Autodesk Fusion 360 part; units mm, degrees
(part 3 of 6)
sketch "Servo Holder" plane through (0, 0, 0) normal (0, 0, -1) x (1, 0, 0)
  line L0 (113.5, 9) -> (83.5, 9)
  line L1 (83.5, 9) -> (83.5, 39)
  line L2 (83.5, 39) -> (33.5, 39)
  arc A0 (33.5, 39) -> (18.5, 24) centre (33.5, 24) ccw
  arc A1 (18.5, 24) -> (22.1849, 0) centre (98.5, 24) ccw
  line L3 (22.1849, 0) -> (0, 0)
  line L4 (0, 0) -> (0, -76)
  line L5 (0, -76) -> (120, -76)
  line L6 (120, -76) -> (120, 0)
  line L7 (120, 0) -> (113.5, 0)
  line L8 (113.5, 0) -> (113.5, 9)
  circle A2 centre (32.5, 24) radius 9
  line L9 (120, 0) -> (79.5, 0)
  line L10 (79.5, 0) -> (79.5, 39)
  line L11 (79.5, 39) -> (120, 39)
  line L12 (120, 39) -> (120, 0)
  dimension "d192" = 40.5
  constraint horizontal L9
  constraint vertical L10
  constraint horizontal L11
  constraint vertical L12
  constraint coincident L6.end L7.start
  constraint collinear L2 L11
  measures "d192" distance of L10.end L11.end
extrude "Extrude46" add sketch "Servo Holder" along normal blind 29 contours L0 L1 L2 L8 L9 L10 L11 | L0 L1 L7 L8 L9 L11 L12
extrude "Extrude50" add 1 faces at (105.6667, -29, 0) along direction (0, 0, 1) blind 4
sketch "Servo Seat" plane through (0, 0, 4) normal (0, 0, 1) x (-1, 0, 0)
  line L0 (-113.5, -41) -> (-113.5, 9)
  line L1 (-113.5, 9) -> (-83.5, 9)
  line L2 (-83.5, 9) -> (-83.5, 39)
  line L3 (-83.5, 39) -> (-120, 39)
  line L4 (-120, 39) -> (-120, -76)
  line L5 (-120, -76) -> (0, -76)
  line L6 (0, -76) -> (0, 0)
  line L7 (0, 0) -> (-22.1849, 0)
  arc A0 (-98.5, -56) -> (-22.1849, 0) centre (-98.5, 24) ccw
  arc A1 (-113.5, -41) -> (-98.5, -56) centre (-98.5, -41) ccw
  line L8 (-83.5, 9) -> (-120, 9)
  line L9 (-120, 9) -> (-120, 18.5)
  line L10 (-120, 18.5) -> (-83.5, 18.5)
  line L11 (-83.5, 18.5) -> (-83.5, 9)
  line L12 (-83.5, 39) -> (-120, 39)
  line L13 (-120, 39) -> (-120, 30.5)
  line L14 (-120, 30.5) -> (-83.5, 30.5)
  line L15 (-83.5, 30.5) -> (-83.5, 39)
  line L16 (-120, 18.5) -> (-115, 18.5)
  line L17 (-115, 18.5) -> (-115, 30.5)
  line L18 (-115, 30.5) -> (-120, 30.5)
  line L19 (-120, 30.5) -> (-120, 18.5)
  line L20 (-113.5, 9) -> (-113.5, 18.5)
  line L21 (-113.5, 30.5) -> (-113.5, 39)
  dimension "d208" = 9.5
  dimension "d211" = 5
  dimension "d225" = 12
  dimension "d226" = 8.5
  dimension "d227" = 6.5
  constraint horizontal L8
  constraint vertical L9
  constraint horizontal L10
  constraint vertical L11
  constraint coincident L1.end L2.start
  constraint horizontal L12
  constraint vertical L13
  constraint horizontal L14
  constraint vertical L15
  constraint coincident L2.end L3.start
  constraint coincident L4 L9.end
  constraint horizontal L16
  constraint vertical L17
  constraint horizontal L18
  constraint vertical L19
  constraint coincident L14 L17.end
  constraint coincident L0.end L1.start
  constraint coincident L10 L20.end
  constraint perpendicular L10 L20
  constraint coincident L14 L21.start
  constraint coincident L3 L21.end
  constraint perpendicular L3 L21
  constraint collinear L20 L21
  constraint collinear L9 L13
  measures "d208" distance of L8.end L9.end
  measures "d211" distance of L17 L19
  measures "d225" distance of L9.end L13.end
  measures "d226" distance of L3.end L13.end
  measures "d227" distance of L13 L21
extrude "Extrude51" cut sketch "Servo Seat" against normal blind 13 contours L4 L10 L14 L16 L17 L18 L19
extrude "Extrude52" cut sketch "Servo Seat" against normal blind 4 contours L1 L2 L8 L10 L11 L20 | L2 L3 L12 L14 L15 L21
extrude "Extrude53" cut sketch "Servo Seat" against normal blind 29 contours L2 L10 L14 L17
sketch "Servo Wires Hole" plane through (79.5, 0, 0) normal (-1, 0, 0) x (0, -1, 0)
  line L0 (39, 0) -> (0, 0)
  line L1 (0, 0) -> (0, -29)
  line L2 (0, -29) -> (39, -29)
  line L3 (39, -29) -> (39, 0)
  line L4 (18.5, -15) -> (30.5, -15)
  line L5 (30.5, -15) -> (30.5, -25)
  line L6 (30.5, -25) -> (18.5, -25)
  line L7 (18.5, -25) -> (18.5, -15)
  dimension "d219" = 8.5
  dimension "d220" = 4
  dimension "d221" = 10
  dimension "d228" = 12
  constraint horizontal L4
  constraint vertical L5
  constraint horizontal L6
  constraint vertical L7
  measures "d219" distance of L3 L5
  measures "d220" distance of L2 L6
  measures "d221" distance of L4.end L5.end
  measures "d228" distance of L5.end L6.end
extrude "Extrude54" cut sketch "Servo Wires Hole" against normal blind 4 contours L4 L5 L6 L7
named bodies: "Colour Detection Mechanism Platform"

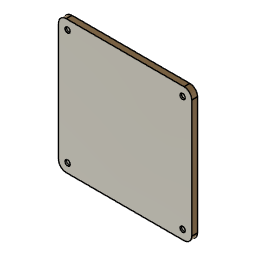
design "Bottom Access Panel"
Autodesk Fusion 360 part; units mm, degrees
sketch "Bottom Access Panel" plane through (0, 0, 0) normal (0, 1, 0) x (1, 0, 0)
  line L0 (0, 0) -> (139, 0)
  line L1 (139, 0) -> (139, -139)
  line L2 (139, -139) -> (0, -139)
  line L3 (0, -139) -> (0, 0)
  dimension "d1" = 139
  dimension "d2" = 139
  constraint horizontal L0
  constraint vertical L1
  constraint horizontal L2
  constraint vertical L3
  constraint coincident L0.start L3.end
  measures "d1" distance of L0.start L0.end
  measures "d2" distance of L0.end L1.end
extrude "Extrude1" add sketch "Bottom Access Panel" along normal blind 6
fillet "Fillet1" radius 8 4 edges at (0, 3, 139) (139, 3, 139) (139, 3, 0) (0, 3, 0)
sketch "Magnet Holes" plane through (0, 0, 0) normal (0, 1, 0) x (1, 0, 0)
  arc A0 (8, 0) -> (0, -8) centre (8, -8) ccw
  line L0 (8, 0) -> (131, 0)
  arc A1 (139, -8) -> (131, 0) centre (131, -8) ccw
  line L1 (139, -8) -> (139, -131)
  arc A2 (131, -139) -> (139, -131) centre (131, -131) ccw
  line L2 (131, -139) -> (8, -139)
  arc A3 (0, -131) -> (8, -139) centre (8, -131) ccw
  line L3 (0, -131) -> (0, -8)
  circle A4 centre (9.5, -129.5) radius 2.75
  circle A5 centre (129.5, -129.5) radius 2.75
  circle A6 centre (9.5, -9.5) radius 2.75
  circle A7 centre (129.5, -9.5) radius 2.75
  dimension "d20" = 5.5
  dimension "d21" = 5.5
  dimension "d22" = 5.5
  dimension "d23" = 5.5
  dimension "d24" = 9.5
  dimension "d25" = 9.5
  dimension "d26" = 9.5
  dimension "d27" = 9.5
  dimension "d28" = 9.5
  dimension "d29" = 9.5
  dimension "d30" = 9.5
  dimension "d31" = 9.5
  measures "d20" diameter of A4
  measures "d21" diameter of A5
  measures "d22" diameter of A6
  measures "d23" diameter of A7
  measures "d24" distance of L1 A5.centre
  measures "d25" distance of L2 A5.centre
  measures "d26" distance of L3 A4.centre
  measures "d27" distance of L2 A4.centre
  measures "d28" distance of L0 A6.centre
  measures "d29" distance of L3 A6.centre
  measures "d30" distance of L1 A7.centre
  measures "d31" distance of L0 A7.centre
extrude "Extrude3" cut sketch "Magnet Holes" along normal blind 1.5 contours A4 | A5 | A6 | A7
equation "mdfThickness = 6 mm"
equation "d4 = mdfThickness"
equation "filletRadius = 8 mm"
equation "d15 = filletRadius"
named bodies: "Bottom Access Panel"

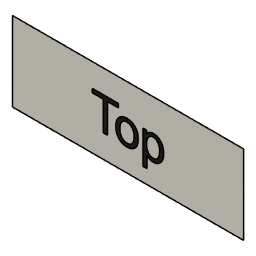
design "Top Label"
part number: 2025-04-13-09-56-45-957
Autodesk Fusion 360 part; units mm, degrees
sketch "Sticker" plane through (0, 0, 0) normal (0, 1, 0) x (1, 0, 0)
  line L0 (0, 0) -> (35, 0)
  line L1 (35, 0) -> (35, -12)
  line L2 (35, -12) -> (0, -12)
  line L3 (0, -12) -> (0, 0)
  dimension "d1" = 35
  dimension "d2" = 12
  constraint horizontal L0
  constraint vertical L1
  constraint horizontal L2
  constraint vertical L3
  constraint coincident L0.start L3.end
  measures "d1" distance of L0.start L0.end
  measures "d2" distance of L0.end L1.end
extrude "Extrude1" add sketch "Sticker" along normal blind 0.01 makes body 1
sketch "Text" plane through (0, 0, 0) normal (0, -1, 0) x (1, 0, 0)
  line L0 (35, 12) -> (0, 12)
  line L1 (0, 12) -> (0, 0)
  line L2 (0, 0) -> (35, 0)
  line L3 (35, 0) -> (35, 12)
  line L4 (0, 0) -> (35, 0) construction
  line L5 (35, 0) -> (35, 12) construction
  line L6 (35, 12) -> (0, 12) construction
  line L7 (0, 12) -> (0, 0) construction
  dimension "d5" = 5
  text T0 "Top" font "Arial" height 5 align centre middle in box 35 x 12 at (0, 0) x (1, 0) y (0, 1) spacing 1 kerned
  constraint coincident L2.end
  constraint coincident L0.end
extrude "Extrude2" add sketch "Text" along normal blind 0.01 separate body text T0 makes body 2 at (19.9566, 0, 4.7193) makes body 3 at (15.8803, 0, 5.5613) makes body 4 at (14.1792, 0, 4.97)
named bodies: "Sticker", "Text 3", "Text 2", "Text 1"

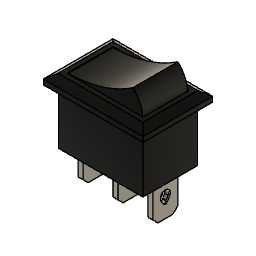
design "Power Switch"
Autodesk Fusion 360 part; units mm, degrees
sketch "Main body" plane through (0, 0, 0) normal (0, 0, 1) x (1, 0, 0)
  line L0 (0, 0) -> (17, 0)
  line L1 (17, 0) -> (17, 11)
  line L2 (17, 11) -> (0, 11)
  line L3 (0, 11) -> (0, 0)
  dimension "d1" = 17
  dimension "d2" = 11
  constraint horizontal L0
  constraint vertical L1
  constraint horizontal L2
  constraint vertical L3
  constraint coincident L0.start L3.end
  measures "d1" distance of L0.start L0.end
  measures "d2" distance of L0.end L1.end
extrude "Extrude1" add sketch "Main body" along normal blind 11 makes body 1
sketch "Top Plate" plane through (0, 0, 11) normal (0, 0, 1) x (-1, 0, 0)
  line L0 (0, -11) -> (0, 0)
  line L1 (0, 0) -> (-17, 0)
  line L2 (-17, 0) -> (-17, -11)
  line L3 (-17, -11) -> (0, -11)
  line L4 (1.5, -12.5) -> (-18.5, -12.5)
  line L5 (-18.5, -12.5) -> (-18.5, 1.5)
  line L6 (-18.5, 1.5) -> (1.5, 1.5)
  line L7 (1.5, 1.5) -> (1.5, -12.5)
  dimension "d5" = 20
  dimension "d6" = 1.5
  dimension "d7" = 1.5
  dimension "d8" = 14
  dimension "d9" = 1.5
  dimension "d10" = 1.5
  constraint horizontal L4
  constraint vertical L5
  constraint horizontal L6
  constraint vertical L7
  measures "d5" distance of L5.end L6.end
  measures "d6" distance of L0 L7
  measures "d7" distance of L2 L5
  measures "d8" distance of L4.end L5.end
  measures "d9" distance of L3 L4
  measures "d10" distance of L1 L6
extrude "Extrude2" add sketch "Top Plate" along normal blind 2 contours L0 L1 L2 L3 | L4 L5 L6 L7 bodies 1
chamfer "Chamfer1" distance 1.5 distance2 1 1 edges at (8.5, -1.5, 13) measured on face at (11.8333, 7.8333, 13) on bodies 1
chamfer "Chamfer1" distance 1.5 distance2 1 3 edges at (18.5, 5.5, 13) (8.5, 12.5, 13) (-1.5, 5.5, 13) measured on face at (11.8333, 7.8333, 13) measured on face at (11.8333, 7.8333, 13) measured on face at (11.8333, 7.8333, 13) on bodies 1
sketch "Switch" plane through (0, 0, 13) normal (0, 0, 1) x (-1, 0, 0)
  line L0 (-17, -11) -> (0, -11)
  line L1 (0, -11) -> (0, 0)
  line L2 (0, 0) -> (-17, 0)
  line L3 (-17, 0) -> (-17, -11)
  line L4 (-1, -10) -> (-16, -10)
  line L5 (-16, -10) -> (-16, -1)
  line L6 (-16, -1) -> (-1, -1)
  line L7 (-1, -1) -> (-1, -10)
  line L8 (-0.9, -10.1) -> (-16.1, -10.1)
  line L9 (-16.1, -10.1) -> (-16.1, -0.9)
  line L10 (-16.1, -0.9) -> (-0.9, -0.9)
  line L11 (-0.9, -0.9) -> (-0.9, -10.1)
  line L12 (-16, -10) -> (-14, -10)
  line L13 (-14, -10) -> (-14, -1)
  line L14 (-14, -1) -> (-16, -1)
  line L15 (-16, -1) -> (-16, -10)
  dimension "d17" = 1
  dimension "d18" = 1
  dimension "d19" = 1
  dimension "d20" = 1
  dimension "d21" = 0.1
  dimension "d22" = 0.1
  dimension "d23" = 0.1
  dimension "d24" = 0.1
  dimension "d29" = 2
  constraint horizontal L4
  constraint vertical L5
  constraint horizontal L6
  constraint vertical L7
  constraint horizontal L8
  constraint vertical L9
  constraint horizontal L10
  constraint vertical L11
  constraint horizontal L12
  constraint vertical L13
  constraint horizontal L14
  constraint vertical L15
  constraint coincident L6 L13.end
  measures "d17" distance of L0 L4
  measures "d18" distance of L2 L6
  measures "d19" distance of L1 L7
  measures "d20" distance of L3 L5
  measures "d21" distance of L4 L8
  measures "d22" distance of L6 L10
  measures "d23" distance of L7 L11
  measures "d24" distance of L5 L9
  measures "d29" distance of L5 L13
extrude "Extrude3" cut sketch "Switch" against normal blind 1 contours L8 L9 L10 L11 bodies 1
extrude "Extrude4" add sketch "Switch" along normal blind 4 contours L4 L5 L6 L12 L13 L14 L15 bodies 1
fillet "Fillet1" radius 6.25 1 edges at (16, 5.5, 17) on bodies 1
fillet "Fillet2" radius 23.5 1 edges at (14, 5.5, 13) on bodies 1
sketch "Pins" plane through (0, 0, 0) normal (0, 0, -1) x (1, 0, 0)
  line L0 (0, 0) -> (0, -11)
  line L1 (0, -11) -> (17, -11)
  line L2 (17, -11) -> (17, 0)
  line L3 (17, 0) -> (0, 0)
  line L4 (1, -8) -> (2, -8)
  line L5 (2, -8) -> (2, -3)
  line L6 (2, -3) -> (1, -3)
  line L7 (1, -3) -> (1, -8)
  line L8 (8, -8) -> (9, -8)
  line L9 (9, -8) -> (9, -3)
  line L10 (9, -3) -> (8, -3)
  line L11 (8, -3) -> (8, -8)
  line L12 (15, -8) -> (16, -8)
  line L13 (16, -8) -> (16, -3)
  line L14 (16, -3) -> (15, -3)
  line L15 (15, -3) -> (15, -8)
  dimension "d34" = 5
  dimension "d37" = 1
  dimension "d38" = 1
  dimension "d39" = 1
  dimension "d40" = 1
  dimension "d41" = 1
  dimension "d42" = 6
  dimension "d43" = 6
  dimension "d44" = 3
  dimension "d45" = 3
  constraint horizontal L4
  constraint vertical L5
  constraint horizontal L6
  constraint vertical L7
  constraint horizontal L8
  constraint vertical L9
  constraint horizontal L10
  constraint vertical L11
  constraint horizontal L12
  constraint vertical L13
  constraint horizontal L14
  constraint vertical L15
  constraint collinear L6 L10
  constraint collinear L10 L14
  constraint collinear L4 L8
  constraint collinear L8 L12
  measures "d34" distance of L4.start L6.end
  measures "d37" distance of L8.start L8.end
  measures "d38" distance of L4.start L4.end
  measures "d39" distance of L12.start L12.end
  measures "d40" distance of L2 L13
  measures "d41" distance of L0 L7
  measures "d42" distance of L5 L11
  measures "d43" distance of L9 L15
  measures "d44" distance of L3 L6
  measures "d45" distance of L1 L4
extrude "Extrude5" add sketch "Pins" along normal blind 7 separate body contours L4 L5 L6 L7 | L8 L9 L10 L11 | L12 L13 L14 L15 makes body 2 at (1, 4.6667, -2.3333) makes body 3 at (8, 4.6667, -2.3333) makes body 4 at (15, 4.6667, -2.3333)
chamfer "Chamfer2" distance 1 angle 45 6 edges at (1.5, 3, -7) (1.5, 8, -7) (15.5, 3, -7) (15.5, 8, -7) (8.5, 3, -7) (8.5, 8, -7) on bodies 2 3 4
sketch "Right Pin Hole" plane through (16, 0, 0) normal (1, 0, 0) x (0, 1, 0)
  line L0 (7, -7) -> (8, -6)
  line L1 (8, -6) -> (8, 0)
  line L2 (8, 0) -> (3, 0)
  line L3 (3, 0) -> (3, -6)
  line L4 (3, -6) -> (4, -7)
  line L5 (4, -7) -> (7, -7)
  circle A0 through (6.4999, -3, -0.005) (5.0001, -2.134, 0.0218) (5, -3.866, 0.0089)
  circle A1 through (6.0012, -4, -0.0057) (5.2512, -3.567, 0.0077) (5.2512, -4.433, 0.0013)
  line L6 (5.9345, -4.2494, -0.0066) -> (6.3666, -3.4989, -0.0069)
  line L7 (5.0685, -4.2505, 0.0052) -> (4.6347, -3.5011, 0.0166)
  dimension "d49" = 2
  dimension "d50" = 4
  dimension "d51" = 2.5
  dimension "d52" = 1
sketch "Middle Pine Hole" plane through (9, 0, 0) normal (1, 0, 0) x (0, 1, 0)
  line L0 (7, -7) -> (8, -6)
  line L1 (8, -6) -> (8, 0)
  line L2 (8, 0) -> (3, 0)
  line L3 (3, 0) -> (3, -6)
  line L4 (3, -6) -> (4, -7)
  line L5 (4, -7) -> (7, -7)
  ellipse E0 centre (5.5, -3) end of major axis (5.9789, -2.1221) minor radius 0.9999
  ellipse E1 centre (5.5012, -4) end of major axis (5.7406, -3.561) minor radius 0.4999
  line L6 (5.9345, -4.2494) -> (6.3666, -3.4989)
  line L7 (5.0685, -4.2505) -> (4.6347, -3.5011)
sketch "Left Pin Hole" plane through (2, 0, 0) normal (1, 0, 0) x (0, 1, 0)
  line L0 (7, -7) -> (8, -6)
  line L1 (8, -6) -> (8, 0)
  line L2 (8, 0) -> (3, 0)
  line L3 (3, 0) -> (3, -6)
  line L4 (3, -6) -> (4, -7)
  line L5 (4, -7) -> (7, -7)
  ellipse E0 centre (5.5, -3) end of major axis (5.9789, -2.1221) minor radius 0.9999
  line L6 (5.0685, -4.2505) -> (4.6347, -3.5011)
  ellipse E1 centre (5.5012, -4) end of major axis (5.7406, -3.561) minor radius 0.4999
  line L7 (5.9345, -4.2494) -> (6.3666, -3.4989)
extrude "Extrude6" cut sketch "Left Pin Hole" against normal blind 1 contours E0 E1 | E0 L6 E1 | E0 E1 L7 | E0 E1 | E0 E1 bodies 2
extrude "Extrude7" cut sketch "Middle Pine Hole" against normal blind 1 contours E0 E1 | E0 E1 L7 | E0 E1 L6 | E0 E1 | E0 E1 bodies 3
extrude "Extrude8" cut sketch "Right Pin Hole" against normal blind 1 contours A0 A1 | A0 A1 L7 | A0 A1 L6 | A0 A1 | A0 A1 in plane through (16.1055, 0.0014, -0.0008) normal (0.99988, 0.01358, -0.007407) bodies 4
equation "d6 = ( ( 20 - 17 ) / 2 ) * 1 mm"
equation "d9 = ( ( 14 - 11 ) / 2 ) * 1 mm"
equation "d44 = ( ( 11 - 5 ) / 2 ) * 1 mm"
named bodies: "Main Body", "Left Pin", "Middle Pin", "Right Pin"

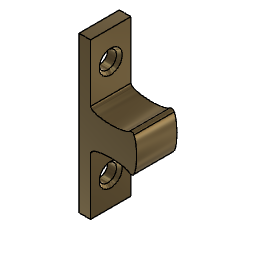
design "Clip Connector Clip"
Autodesk Fusion 360 part; units mm, degrees
sketch "Sketch1" plane through (0, 0, 0) normal (1, 0, 0) x (0, 1, 0)
  line L0 (0, 0) -> (7, 0)
  line L1 (7, 0) -> (7, 27)
  line L2 (7, 27) -> (0, 27)
  line L3 (0, 27) -> (0, 0)
  dimension "d1" = 7
  dimension "d2" = 27
  constraint horizontal L0
  constraint vertical L1
  constraint horizontal L2
  constraint vertical L3
  constraint coincident L0.start L3.end
  measures "d1" distance of L1.end L2.end
  measures "d2" distance of L0.end L1.end
extrude "Extrude1" add sketch "Sketch1" along normal blind 2
sketch "Sketch2" plane through (2, 0, 0) normal (1, 0, 0) x (0, 1, 0)
  line L0 (0, 27) -> (0, 0)
  line L1 (0, 0) -> (7, 0)
  line L2 (7, 0) -> (7, 27)
  line L3 (7, 27) -> (0, 27)
  line L4 (0, 17) -> (7, 17)
  line L5 (7, 17) -> (7, 10)
  line L6 (7, 10) -> (0, 10)
  line L7 (0, 10) -> (0, 17)
  circle A0 centre (3.5, 22) radius 1.5
  circle A1 centre (3.5, 5) radius 1.5
  dimension "d5" = 3.5
  dimension "d6" = 3.5
  dimension "d7" = 3
  dimension "d8" = 3
  dimension "d9" = 7
  dimension "d10" = 10
  dimension "d11" = 10
  dimension "d12" = 5
  dimension "d13" = 5
  dimension "d33" = 5
  dimension "d34" = 5
  constraint horizontal L4
  constraint vertical L5
  constraint horizontal L6
  constraint vertical L7
  constraint coincident L2 L5.end
  constraint coincident L0 L4.start
  measures "d5" distance of L0 A0.centre
  measures "d6" distance of L0 A1.centre
  measures "d7" diameter of A0
  measures "d8" diameter of A1
  measures "d9" distance of L4 L6
  measures "d10" distance of L3 L4
  measures "d11" distance of L1 L6
  measures "d12" distance of L3 A0.centre
  measures "d13" distance of L1 A1.centre
  measures "d33" distance of L4 A0.centre
  measures "d34" distance of L6 A1.centre
extrude "Extrude2" cut sketch "Sketch2" against normal blind 2 contours A0 | A1
chamfer "Chamfer1" distance 0.5 angle 45 2 edges at (2, 2.1015, 22.5424) (2, 2.1015, 5.5424)
extrude "Extrude3" add sketch "Sketch2" along normal blind 7 contours L0 L2 L4 L5 L6 L7
sketch "Sketch4" plane through (0, 0, 0) normal (0, -1, 0) x (1, 0, 0)
  line L0 (0, 27) -> (0, 0)
  line L1 (0, 0) -> (2, 0)
  line L2 (2, 0) -> (2, 10)
  line L3 (2, 10) -> (9, 10)
  line L4 (9, 10) -> (9, 17)
  line L5 (9, 17) -> (2, 17)
  line L6 (2, 17) -> (2, 27)
  line L7 (2, 27) -> (0, 27)
  ellipse E0 centre (9, 13.5) end of major axis (9, 17) minor radius 1
  line L8 (9, 10) -> (9, 17)
  line L9 (10, 13.5) -> (8, 13.5)
  dimension "d35" = 2
  constraint coincident L3.end E0
  constraint coincident L4.end E0
  constraint coincident E0 L9.start
  constraint coincident E0 L9.end
extrude "Extrude5" add sketch "Sketch4" against normal blind 7 contours L4 E0 L8 L9 | L4 E0 L8 L9 picked at (9.6303, 14.0297) picked at (9.2475, 11.5518)
sketch "Sketch5" plane through (0, 0, 0) normal (0, -1, 0) x (1, 0, 0)
  line L0 (0, 27) -> (0, 0)
  line L1 (0, 0) -> (2, 0)
  line L2 (2, 0) -> (2, 10)
  line L3 (2, 10) -> (9, 10)
  line L4 (9, 17) -> (2, 17)
  line L5 (2, 17) -> (2, 27)
  line L6 (2, 27) -> (0, 27)
  ellipse E0 centre (9, 13.5) end of major axis (9, 17) minor radius 1 (9, 10) -> (9, 17) ccw
  ellipse E1 centre (5.5, 17) end of major axis (9, 17) minor radius 1
  line L7 (2, 17) -> (9, 17)
  line L8 (5.5, 16) -> (5.5, 18)
  ellipse E2 centre (5.5, 10) end of major axis (9, 10) minor radius 1
  line L9 (2, 10) -> (9, 10)
  line L10 (5.5, 9) -> (5.5, 11)
  dimension "d36" = 2
  dimension "d37" = 2
  constraint coincident L4.end E1
  constraint coincident L4.start E1
  constraint coincident E1 L8.start
  constraint coincident E1 L8.end
  constraint coincident L4 E1.centre
  constraint coincident E2 L2.end
  constraint coincident L3.end E2
  constraint coincident E2 L10.start
  constraint coincident E2 L10.end
  constraint coincident L3 E2.centre
  constraint coincident L4.end L5.start
extrude "Extrude6" cut sketch "Sketch5" against normal blind 7 contours L4 E1 L7 L8 | L3 E2 L9 L10 | L4 E1 L7 L8 | L3 E2 L9 L10 picked at (3.5518, 16.7525) picked at (4.9703, 10.6303) picked at (6.0297, 16.3697) picked at (7.4482, 10.2475)
fillet "Fillet2" radius 0.5 2 edges at (9, 3.5, 17) (9, 3.5, 10)
equation "d5 = ( 7 / 2 ) * 1 mm"
equation "d6 = ( 7 / 2 ) * 1 mm"
equation "d10 = ( ( 27 - 7 ) / 2 ) * 1 mm"
equation "d12 = ( 10 / 2 ) * 1 mm"
equation "d13 = ( 10 / 2 ) * 1 mm"
named bodies: "Clip Connector Clip"

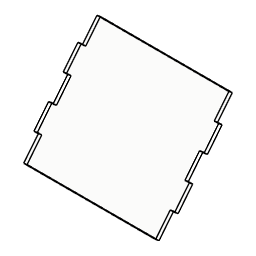
design "Slide Panel"
part number: 2025-05-20-12-54-31-195
Autodesk Fusion 360 part; units mm, degrees
sketch "Slide" plane through (0, 0, 0) normal (1, 0, 0) x (0, 1, 0)
  line L0 (0, 0) -> (49.9812, 62.4765)
  line L1 (49.9812, 62.4765) -> (52.3238, 60.6024)
  line L2 (0, 0) -> (2.3426, -1.8741)
  line L3 (2.3426, -1.8741) -> (52.3238, 60.6024)
  dimension "d2" = 80.009
  dimension "d3" = 3
  dimension "d4" = 3
  constraint coincident L0.start L2.start
  constraint perpendicular L0 L1
  constraint perpendicular L0 L2
  measures "d2" distance of L0.start L0.end
  measures "d3" distance of L0.end L1.end
  measures "d4" distance of L0.start L2.end
extrude "Extrude1" add sketch "Slide" against normal blind 96
sketch "Top" plane through (0, 0, 0) normal (0, -0.780869, 0.624695) x (1, 0, 0)
  line L0 (0, 0) -> (0, 80.009)
  line L1 (0, 80.009) -> (-96, 80.009)
  line L2 (-96, 80.009) -> (-96, 0)
  line L3 (-96, 0) -> (0, 0)
  line L4 (0, 80.009) -> (-3, 80.009)
  line L5 (-3, 80.009) -> (-3, 64.009)
  line L6 (-3, 64.009) -> (0, 64.009)
  line L7 (0, 64.009) -> (0, 80.009)
  line L8 (0, 48.009) -> (-3, 48.009)
  line L9 (-3, 48.009) -> (-3, 32.009)
  line L10 (-3, 32.009) -> (0, 32.009)
  line L11 (0, 32.009) -> (0, 48.009)
  line L12 (0, 16) -> (-3, 16)
  line L13 (-3, 16) -> (-3, 0)
  line L14 (-3, 0) -> (0, 0)
  line L15 (0, 0) -> (0, 16)
  line L16 (-96, 80.009) -> (-93, 80.009)
  line L17 (-93, 80.009) -> (-93, 64.009)
  line L18 (-93, 64.009) -> (-96, 64.009)
  line L19 (-96, 64.009) -> (-96, 80.009)
  line L20 (-96, 48.009) -> (-93, 48.009)
  line L21 (-93, 48.009) -> (-93, 32.009)
  line L22 (-93, 32.009) -> (-96, 32.009)
  line L23 (-96, 32.009) -> (-96, 48.009)
  line L24 (-96, 16) -> (-93, 16)
  line L25 (-93, 16) -> (-93, 0)
  line L26 (-93, 0) -> (-96, 0)
  line L27 (-96, 0) -> (-96, 16)
  dimension "d7" = 3
  dimension "d8" = 16
  dimension "d9" = 16
  dimension "d10" = 16
  dimension "d11" = 16
  dimension "d12" = 16.009
  dimension "d13" = 3
  dimension "d14" = 16
  dimension "d15" = 16
  dimension "d16" = 16
  dimension "d17" = 16
  dimension "d18" = 16.009
  constraint horizontal L4
  constraint vertical L5
  constraint horizontal L6
  constraint vertical L7
  constraint coincident L0.end L1.start
  constraint horizontal L8
  constraint vertical L9
  constraint horizontal L10
  constraint vertical L11
  constraint coincident L0 L8.start
  constraint horizontal L12
  constraint vertical L13
  constraint horizontal L14
  constraint vertical L15
  constraint coincident L3 L13.end
  constraint coincident L0 L12.start
  constraint collinear L5 L9
  constraint collinear L9 L13
  constraint horizontal L16
  constraint vertical L17
  constraint horizontal L18
  constraint vertical L19
  constraint coincident L1.end L2.start
  constraint horizontal L20
  constraint vertical L21
  constraint horizontal L22
  constraint vertical L23
  constraint coincident L2 L20.start
  constraint horizontal L24
  constraint vertical L25
  constraint horizontal L26
  constraint vertical L27
  constraint coincident L3 L25.end
  constraint coincident L2 L24.start
  constraint collinear L17 L21
  constraint collinear L21 L25
  measures "d7" distance of L5 L7
  measures "d8" distance of L0.end L6.end
  measures "d9" distance of L8.start L10.end
  measures "d10" distance of L6 L8
  measures "d11" distance of L12.start L0.start
  measures "d12" distance of L10 L12
  measures "d13" distance of L1.end L16.end
  measures "d14" distance of L1.end L18.end
  measures "d15" distance of L20.start L22.end
  measures "d16" distance of L24.start L2.end
  measures "d17" distance of L18 L20
  measures "d18" distance of L22 L24
extrude "Extrude2" cut sketch "Top" against normal blind 3 contours L0 L3 L12 L13 L14 L15 | L0 L8 L9 L10 L11 | L2 L3 L24 L25 L26 L27 | L0 L1 L4 L5 L6 L7 | L2 L20 L21 L22 L23 | L1 L2 L16 L17 L18 L19
equation "acrylic_thickness = 3 mm"
equation "d3 = acrylic_thickness"
equation "d4 = acrylic_thickness"
equation "d7 = acrylic_thickness"
equation "d13 = acrylic_thickness"
named bodies: "Slide Panel"

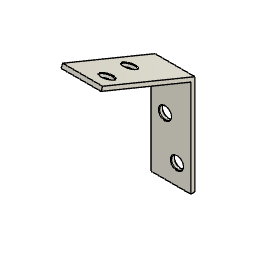
design "Top Panel Connector"
Autodesk Fusion 360 part; units mm, degrees
sketch "Sketch1" plane through (0, 0, 0) normal (1, 0, 0) x (0, 1, 0)
  line L0 (0, 0) -> (0, 50)
  line L1 (0, 50) -> (-46.2605, 68.9728)
  line L2 (-46.2605, 68.9728) -> (-47.0194, 67.1224)
  line L3 (-47.0194, 67.1224) -> (-2, 48.6586)
  line L4 (-2, 48.6586) -> (-2, 0)
  line L5 (-2, 0) -> (0, 0)
  dimension "d1" = 2
  dimension "d2" = 2
  dimension "d3" = 50
  dimension "d4" = 50
  dimension "d27" = 112.3
  constraint coincident L0.start L5.end
  constraint vertical L0
  constraint perpendicular L1 L2
  constraint perpendicular L2 L3
  constraint vertical L4
  constraint perpendicular L0 L5
  measures "d1" distance of L1.end L2.end
  measures "d2" distance of L4.end L0.start
  measures "d3" distance of L0.start L0.end
  measures "d4" distance of L0.end L1.end
  measures "d27" angle of L3 L4
extrude "Extrude1" add sketch "Sketch1" against normal blind 20
sketch "Sketch2" plane through (0, -2, 0) normal (0, -1, 0) x (1, 0, 0)
  line L0 (0, 0) -> (0, 48.6586)
  line L1 (0, 48.6586) -> (-20, 48.6586)
  line L2 (-20, 48.6586) -> (-20, 0)
  line L3 (-20, 0) -> (0, 0)
  circle A0 centre (-13, 28.6586) radius 3
  circle A1 centre (-7, 10) radius 3
  point P0 (0, 50)
  dimension "d7" = 10
  dimension "d8" = 20
  dimension "d10" = 18.6586
  dimension "d11" = 7
  dimension "d12" = 7
  dimension "d13" = 6
  dimension "d14" = 6
  measures "d7" distance of L3 A1.centre
  measures "d8" distance of L1 A0.centre
  measures "d10" distance of A0.centre A1.centre
  measures "d11" distance of L2 A0.centre
  measures "d12" distance of L0 A1.centre
  measures "d13" diameter of A0
  measures "d14" diameter of A1
sketch "Sketch3" plane through (0, 16.7949, 40.9502) normal (0, -0.379456, -0.92521) x (1, 0, 0)
  line L0 (0, 20.3142) -> (0, 68.9728)
  line L1 (0, 68.9728) -> (-20, 68.9728)
  line L2 (-20, 68.9728) -> (-20, 20.3142)
  line L3 (-20, 20.3142) -> (0, 20.3142)
  circle A0 centre (-7, 58.9728) radius 3
  circle A1 centre (-13, 40.3142) radius 3
  line L4 (0, 20.3142) -> (-20, 20.3142)
  dimension "d15" = 6
  dimension "d16" = 6
  dimension "d17" = 7
  dimension "d18" = 7
  dimension "d19" = 10
  dimension "d20" = 20
  dimension "d28" = 18.6586
  measures "d15" diameter of A0
  measures "d16" diameter of A1
  measures "d17" distance of L0 A0.centre
  measures "d18" distance of L2 A1.centre
  measures "d19" distance of L1 A0.centre
  measures "d20" distance of A1.centre L4
  measures "d28" distance of A0.centre A1.centre
extrude "Extrude2" cut sketch "Sketch3" against normal blind 2 contours A0 | A1
extrude "Extrude3" cut sketch "Sketch2" against normal blind 2 contours A0 | A1
fillet "Fillet1" radius 0.3 8 edges at (-9.797, -38.771, 63.7395) (-15.797, -21.5079, 56.6594) (-15.797, -2, 29.7434) (-9.797, -2, 11.0848) (-9.797, 0, 8.9152) (-15.797, 0, 27.5737) (-9.797, -36.0047, 64.7666) (-15.797, -18.7416, 57.6865)
named bodies: "Top Panel and Back Panel Connector"

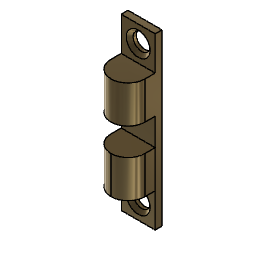
design "Clip Connector Base"
Autodesk Fusion 360 part; units mm, degrees
sketch "Sketch1" plane through (0, 0, 0) normal (0, 1, 0) x (1, 0, 0)
  line L0 (0, 0) -> (10, 0)
  line L1 (10, 0) -> (10, -50)
  line L2 (10, -50) -> (0, -50)
  line L3 (0, -50) -> (0, 0)
  dimension "d1" = 10
  dimension "d2" = 50
  constraint horizontal L0
  constraint vertical L1
  constraint horizontal L2
  constraint vertical L3
  constraint coincident L0.start L3.end
  measures "d1" distance of L1.end L2.end
  measures "d2" distance of L0.end L1.end
extrude "Extrude1" add sketch "Sketch1" against normal blind 2
sketch "Sketch2" plane through (0, -2, 0) normal (0, -1, 0) x (1, 0, 0)
  line L0 (10, 50) -> (0, 50)
  line L1 (0, 50) -> (0, 0)
  line L2 (0, 0) -> (10, 0)
  line L3 (10, 0) -> (10, 50)
  line L4 (0, 40) -> (10, 40)
  line L5 (10, 40) -> (10, 29)
  line L6 (10, 29) -> (0, 29)
  line L7 (0, 29) -> (0, 40)
  line L8 (0, 10) -> (10, 10)
  line L9 (10, 10) -> (10, 21)
  line L10 (10, 21) -> (0, 21)
  line L11 (0, 21) -> (0, 10)
  circle A0 centre (5, 45) radius 2.5
  circle A1 centre (5, 5) radius 2.5
  dimension "d5" = 5
  dimension "d6" = 5
  dimension "d7" = 5
  dimension "d8" = 5
  dimension "d9" = 11
  dimension "d10" = 11
  dimension "d11" = 10
  dimension "d12" = 10
  dimension "d13" = 8
  dimension "d14" = 5
  dimension "d15" = 5
  dimension "d16" = 5
  constraint horizontal L4
  constraint vertical L5
  constraint horizontal L6
  constraint vertical L7
  constraint coincident L3 L5.end
  constraint coincident L1 L4.start
  constraint horizontal L8
  constraint vertical L9
  constraint horizontal L10
  constraint vertical L11
  constraint coincident L3 L9.end
  constraint coincident L1 L8.start
  measures "d5" distance of L1 A0.centre
  measures "d6" distance of L1 A1.centre
  measures "d7" diameter of A1
  measures "d8" diameter of A0
  measures "d9" distance of L4.end L5.end
  measures "d10" distance of L8.end L9.end
  measures "d11" distance of L0 L4
  measures "d12" distance of L2 L8
  measures "d13" distance of L6 L10
  measures "d14" distance of L4 A0.centre
  measures "d15" distance of L2 A1.centre
  measures "d16" distance of L8 A1.centre
extrude "Extrude2" add sketch "Sketch2" along normal blind 8 contours L1 L3 L4 L5 L6 L7 | L1 L3 L8 L9 L10 L11
extrude "Extrude3" cut sketch "Sketch2" against normal blind 2 contours A0 | A1
chamfer "Chamfer1" distance 1 angle 45 2 edges at (2.6692, -2, 45.904) (2.6692, -2, 5.904)
fillet "Fillet1" radius 5 4 edges at (0, -10, 34.5) (0, -10, 15.5) (10, -10, 34.5) (10, -10, 15.5)
named bodies: "Clip Connector Base"

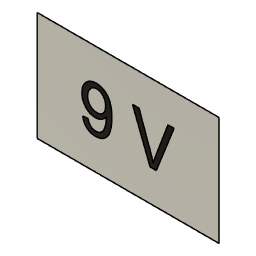
design "9 Volt Label"
part number: 2025-04-13-10-20-13-952
Autodesk Fusion 360 part; units mm, degrees
sketch "Sticker" plane through (0, 0, 0) normal (0, 1, 0) x (1, 0, 0)
  line L0 (0, 0) -> (20, 0)
  line L1 (20, 0) -> (20, -12)
  line L2 (20, -12) -> (0, -12)
  line L3 (0, -12) -> (0, 0)
  dimension "d1" = 12
  dimension "d2" = 20
  constraint horizontal L0
  constraint vertical L1
  constraint horizontal L2
  constraint vertical L3
  constraint coincident L0.start L3.end
  measures "d1" distance of L0.end L1.end
  measures "d2" distance of L0.start L0.end
extrude "Extrude1" add sketch "Sticker" along normal blind 0.01 makes body 1
sketch "Text" plane through (0, 0, 0) normal (0, -1, 0) x (1, 0, 0)
  line L0 (20, 12) -> (0, 12)
  line L1 (0, 12) -> (0, 0)
  line L2 (0, 0) -> (20, 0)
  line L3 (20, 0) -> (20, 12)
  line L4 (0, 0) -> (20, 0) construction
  line L5 (20, 0) -> (20, 12) construction
  line L6 (20, 12) -> (0, 12) construction
  line L7 (0, 12) -> (0, 0) construction
  dimension "d5" = 5
  text T0 "9 V" font "Arial" height 5 align centre middle in box 20 x 12 at (0, 0) x (1, 0) y (0, 1) spacing 1 kerned
  constraint coincident L2.end
  constraint coincident L0.end
extrude "Extrude2" add sketch "Text" along normal blind 0.01 separate body text T0 makes body 2 at (8.0045, 0, 5.7492) makes body 3 at (11.4069, 0, 7.2892)
named bodies: "Sticker", "Text 1", "Text 2"

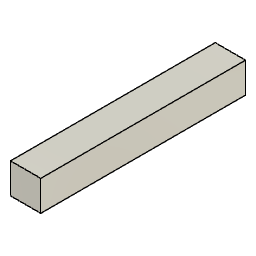
design "Sorted Smarties Top Support Left"
Autodesk Fusion 360 part; units mm, degrees
sketch "Back Panel Support Left " plane through (0, 0, 0) normal (1, 0, 0) x (0, 1, 0)
  line L0 (0, 0) -> (142, 0)
  line L1 (142, 0) -> (142, 21)
  line L2 (142, 21) -> (0, 21)
  line L3 (0, 21) -> (0, 0)
  dimension "d1" = 21
  dimension "d2" = 142
  constraint horizontal L0
  constraint vertical L1
  constraint horizontal L2
  constraint vertical L3
  constraint coincident L0.start L3.end
  measures "d1" distance of L0.end L1.end
  measures "d2" distance of L0.start L0.end
extrude "Extrude1" add sketch "Back Panel Support Left " along normal blind 21
named bodies: "Sorted Smarties Top Support Left"

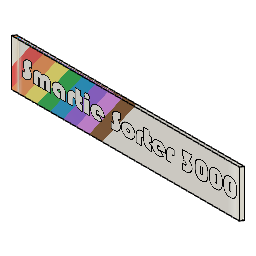
design "Name Sign"
Autodesk Fusion 360 part; units mm, degrees
sketch "Name Sign" plane through (0, 0, 0) normal (1, 0, 0) x (0, 1, 0) in component "Name Sign"
  line L0 (-0.0158, 97.2466) -> (5.9842, 94.7858)
  line L1 (5.9842, 150.2078) -> (-0.0158, 152.6686)
  line L2 (-0.0158, 152.6686) -> (-0.0158, 97.2466)
  line L3 (5.9842, 150.2078) -> (5.9842, 94.7858)
  dimension "d18" = 67.7
  dimension "d8" = 6
  dimension "d9" = 55.422
  constraint vertical L2
  constraint parallel L2 L3
  measures "d18" angle of L0 L3
  measures "d8" distance of L2 L3
  measures "d9" distance of L1.end L0.start
extrude "Extrude2" add sketch "Name Sign" along normal blind 270 in component "Name Sign"
component "Name Sign" placed x (1, 0, 0) y (0, 1, 0) z (0, 0, 1) at (0, 0, 0)
equation "polycarbonateThickness = 6 mm"
named bodies: "Name Sign"

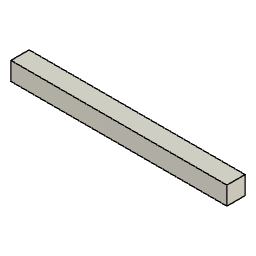
design "Back Panel Support Middle"
Autodesk Fusion 360 part; units mm, degrees
sketch "Back Panel Support Left " plane through (0, 0, 0) normal (1, 0, 0) x (0, 1, 0)
  line L0 (0, 0) -> (21, 0)
  line L1 (21, 0) -> (21, 21)
  line L2 (21, 21) -> (0, 21)
  line L3 (0, 21) -> (0, 0)
  dimension "d1" = 21
  dimension "d2" = 21
  constraint horizontal L0
  constraint vertical L1
  constraint horizontal L2
  constraint vertical L3
  constraint coincident L0.start L3.end
  measures "d1" distance of L0.end L1.end
  measures "d2" distance of L0.start L0.end
extrude "Extrude1" add sketch "Back Panel Support Left " along normal blind 249
named bodies: "Back Panel Support Middle"

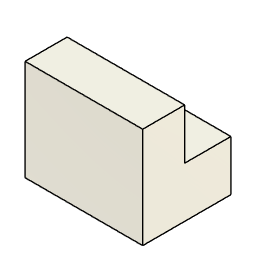
design "Colour Detection Mechanism Top Panel Support"
part number: 2025-05-14-09-44-42-407
Autodesk Fusion 360 part; units mm, degrees
sketch "Sorting Mechanism Top Panel Support" plane through (0, 0, 0) normal (0, 0, 1) x (1, 0, 0)
  line L0 (0, 0) -> (28, 0)
  line L1 (28, 0) -> (28, 10)
  line L2 (28, 10) -> (0, 10)
  line L3 (0, 10) -> (0, 0)
  line L4 (28, 10) -> (0, 10)
  line L5 (0, 10) -> (0, 21)
  line L6 (0, 21) -> (28, 21)
  line L7 (28, 21) -> (28, 10)
  dimension "d1" = 10
  dimension "d2" = 28
  dimension "d5" = 11
  constraint horizontal L0
  constraint vertical L1
  constraint horizontal L2
  constraint vertical L3
  constraint coincident L0.start L3.end
  constraint horizontal L4
  constraint vertical L5
  constraint horizontal L6
  constraint vertical L7
  constraint collinear L3 L5
  measures "d1" distance of L0.end L1.end
  measures "d2" distance of L0.start L0.end
  measures "d5" distance of L1.end L6.end
extrude "Extrude1" add sketch "Sorting Mechanism Top Panel Support" along normal blind 24 contours L0 L1 L2 L3 L4
extrude "Extrude2" add sketch "Sorting Mechanism Top Panel Support" along normal blind 12 contours L2 L4 L5 L6 L7
named bodies: "Sorting Mechanism Top Panel Support"

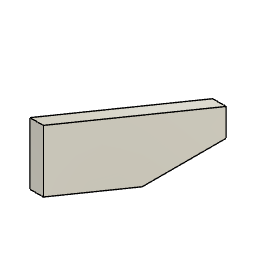
design "Name Sign Support Left"
Autodesk Fusion 360 part; units mm, degrees
sketch "Name Sign Support" plane through (0, 0, 0) normal (1, 0, 0) x (0, 1, 0) in component "Name Sign Support (1)"
  line L0 (-0.0158, 97.2466) -> (88.3556, 61.0028)
  line L1 (163.2949, 85.69) -> (-0.0158, 152.6686)
  line L2 (-0.0158, 152.6686) -> (-0.0158, 97.2466)
  line L3 (163.2949, 85.69) -> (163.2949, 61.0028)
  line L4 (88.3556, 61.0028) -> (163.2949, 61.0028)
  dimension "d18" = 67.7
  dimension "d9" = 55.422
  dimension "d2" = 176.512
  dimension "d3" = 95.515
  constraint vertical L2
  constraint parallel L2 L3
  constraint perpendicular L3 L4
  measures "d18" angle of L0 L3
  measures "d9" distance of L1.end L0.start
  measures "d2" distance of L1.start L1.end
  measures "d3" distance of L0.start L0.end
extrude "Extrude2" add sketch "Name Sign Support" along normal blind 12 in component "Name Sign Support (1)"
component "Name Sign Support Left" placed x (1, 0, 0) y (0, 1, 0) z (0, 0, 1) at (0, 0, 0)
component "Name Sign Support" placed x (1, 0, 0) y (0, 1, 0) z (0, 0, 1) at (0, 0, 0) in component "Name Sign Support Left"
component "Name Sign Support (1)" placed x (1, 0, 0) y (0, 1, 0) z (0, 0, 1) at (0, 0, 0) in component "Name Sign Support"
equation "d19 = pineThickness"
equation "pineThickness = 12 mm"
named bodies: "Name Sign Support"

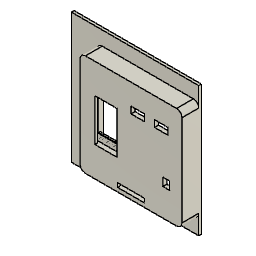
design "Electronics Holder"
Autodesk Fusion 360 part; units mm, degrees
sketch "Sketch1" plane through (0, 0, 0) normal (0, 1, 0) x (1, 0, 0)
  line L0 (0, 0) -> (190, 0)
  line L1 (190, 0) -> (190, -194)
  line L2 (190, -194) -> (0, -194)
  line L3 (0, -194) -> (0, 0)
  dimension "d1" = 190
  dimension "d2" = 194
  constraint horizontal L0
  constraint vertical L1
  constraint horizontal L2
  constraint vertical L3
  constraint coincident L0.start L3.end
  measures "d1" distance of L0.start L0.end
  measures "d2" distance of L0.end L1.end
extrude "Extrude1" add sketch "Sketch1" against normal blind 4
sketch "Sketch2" plane through (0, -4, 0) normal (0, -1, 0) x (1, 0, 0)
  line L0 (190, 194) -> (0, 194)
  line L1 (0, 194) -> (0, 0)
  line L2 (0, 0) -> (190, 0)
  line L3 (190, 0) -> (190, 194)
  line L4 (44, 167) -> (184, 167)
  line L5 (184, 167) -> (184, 27)
  line L6 (184, 27) -> (44, 27)
  line L7 (44, 27) -> (44, 167)
  dimension "d5" = 44
  dimension "d6" = 140
  dimension "d7" = 27
  dimension "d8" = 140
  constraint horizontal L4
  constraint vertical L5
  constraint horizontal L6
  constraint vertical L7
  measures "d5" distance of L1 L7
  measures "d6" distance of L5.end L6.end
  measures "d7" distance of L2 L6
  measures "d8" distance of L4.end L5.end
extrude "Extrude2" cut sketch "Sketch2" against normal blind 4 contours L4 L5 L6 L7
fillet "Fillet1" radius 8 4 edges at (44, -2, 167) (44, -2, 27) (184, -2, 167) (184, -2, 27)
sketch "Sketch3" plane through (0, -4, 0) normal (0, -1, 0) x (1, 0, 0)
  line L0 (184, 159) -> (184, 35)
  arc A0 (176, 27) -> (184, 35) centre (176, 35) ccw
  line L1 (176, 27) -> (52, 27)
  arc A1 (44, 35) -> (52, 27) centre (52, 35) ccw
  line L2 (44, 35) -> (44, 159)
  arc A2 (52, 167) -> (44, 159) centre (52, 159) ccw
  line L3 (52, 167) -> (176, 167)
  arc A3 (184, 159) -> (176, 167) centre (176, 159) ccw
  line L4 (190, 194) -> (0, 194)
  line L5 (0, 194) -> (0, 0)
  line L6 (0, 0) -> (190, 0)
  line L7 (190, 0) -> (190, 194)
  line L8 (38, 173) -> (190, 173)
  line L9 (190, 173) -> (190, 21)
  line L10 (190, 21) -> (38, 21)
  line L11 (38, 21) -> (38, 173)
  dimension "d13" = 6
  dimension "d14" = 6
  dimension "d15" = 6
  dimension "d16" = 6
  constraint horizontal L8
  constraint vertical L9
  constraint horizontal L10
  constraint vertical L11
  constraint coincident L7 L9.end
  measures "d13" distance of L0 L9
  measures "d14" distance of L2 L11
  measures "d15" distance of L1 L10
  measures "d16" distance of L3 L8
extrude "Extrude3" add sketch "Sketch3" along normal blind 21 contours L7 L8 L9 L10 L11
sketch "Sketch4" plane through (0, -25, 0) normal (0, -1, 0) x (1, 0, 0)
  arc A0 (176, 27) -> (184, 35) centre (176, 35) ccw
  line L0 (176, 27) -> (52, 27)
  arc A1 (44, 35) -> (52, 27) centre (52, 35) ccw
  line L1 (44, 35) -> (44, 159)
  arc A2 (52, 167) -> (44, 159) centre (52, 159) ccw
  line L2 (52, 167) -> (176, 167)
  arc A3 (184, 159) -> (176, 167) centre (176, 159) ccw
  line L3 (184, 159) -> (184, 35)
  line L4 (38, 21) -> (190, 21)
  line L5 (190, 21) -> (190, 173)
  line L6 (190, 173) -> (38, 173)
  line L7 (38, 173) -> (38, 21)
  line L8 (38, 173) -> (190, 173)
  line L9 (190, 173) -> (190, 21)
  line L10 (190, 21) -> (38, 21)
  line L11 (38, 21) -> (38, 173)
  constraint horizontal L8
  constraint vertical L9
  constraint horizontal L10
  constraint vertical L11
  constraint coincident L4.end L5.start
  constraint coincident L6.end L7.start
extrude "Extrude4" add sketch "Sketch4" along normal blind 4 contours A0 L0 A1 L1 A2 L2 A3 L3 | L4 L5 L6 L7 L8 L9 L10 L11
fillet "Fillet2" radius 8 4 edges at (38, -16.5, 173) (190, -16.5, 173) (38, -16.5, 21) (190, -16.5, 21)
sketch "Sketch5" plane through (0, 0, 0) normal (0, 1, 0) x (-1, 0, 0)
  line L0 (-184, 35) -> (-184, 159)
  arc A0 (-176, 167) -> (-184, 159) centre (-176, 159) ccw
  line L1 (-176, 167) -> (-52, 167)
  arc A1 (-44, 159) -> (-52, 167) centre (-52, 159) ccw
  line L2 (-44, 159) -> (-44, 35)
  arc A2 (-52, 27) -> (-44, 35) centre (-52, 35) ccw
  line L3 (-52, 27) -> (-176, 27)
  arc A3 (-184, 35) -> (-176, 27) centre (-176, 35) ccw
  line L4 (0, 194) -> (-190, 194)
  line L5 (-190, 194) -> (-190, 0)
  line L6 (-190, 0) -> (0, 0)
  line L7 (0, 0) -> (0, 194)
  line L8 (-64, 167) -> (-44, 167)
  line L9 (-44, 167) -> (-44, 147)
  line L10 (-44, 147) -> (-64, 147)
  line L11 (-64, 147) -> (-64, 167)
  circle A4 centre (-54, 157) radius 2.75
  line L12 (-164, 167) -> (-184, 167)
  line L13 (-184, 167) -> (-184, 147)
  line L14 (-184, 147) -> (-164, 147)
  line L15 (-164, 147) -> (-164, 167)
  line L16 (-184, 47) -> (-164, 47)
  line L17 (-164, 47) -> (-164, 27)
  line L18 (-164, 27) -> (-184, 27)
  line L19 (-184, 27) -> (-184, 47)
  line L20 (-44, 47) -> (-64, 47)
  line L21 (-64, 47) -> (-64, 27)
  line L22 (-64, 27) -> (-44, 27)
  line L23 (-44, 27) -> (-44, 47)
  circle A5 centre (-174, 157) radius 2.75
  circle A6 centre (-174, 37) radius 2.75
  circle A7 centre (-54, 37) radius 2.75
  dimension "d23" = 5.5
  dimension "d24" = 10
  dimension "d25" = 10
  dimension "d26" = 10
  dimension "d27" = 10
  dimension "d28" = 5.5
  dimension "d29" = 10
  dimension "d30" = 10
  dimension "d31" = 10
  dimension "d32" = 10
  dimension "d33" = 5.5
  dimension "d34" = 5.5
  dimension "d35" = 10
  dimension "d36" = 10
  dimension "d37" = 10
  dimension "d38" = 10
  dimension "d39" = 10
  dimension "d40" = 10
  dimension "d41" = 10
  dimension "d42" = 10
  constraint horizontal L8
  constraint vertical L9
  constraint horizontal L10
  constraint vertical L11
  constraint coincident L2 L9.end
  constraint coincident L1 L8.start
  constraint horizontal L12
  constraint vertical L13
  constraint horizontal L14
  constraint vertical L15
  constraint coincident L0 L13.end
  constraint coincident L1 L12.start
  constraint horizontal L16
  constraint vertical L17
  constraint horizontal L18
  constraint vertical L19
  constraint coincident L3 L17.end
  constraint coincident L0 L16.start
  constraint horizontal L20
  constraint vertical L21
  constraint horizontal L22
  constraint vertical L23
  constraint coincident L3 L21.end
  constraint coincident L2 L20.start
  measures "d23" diameter of A4
  measures "d24" distance of L9 A4.centre
  measures "d25" distance of L8 A4.centre
  measures "d26" distance of L11 A4.centre
  measures "d27" distance of L10 A4.centre
  measures "d28" diameter of A5
  measures "d29" distance of L12 A5.centre
  measures "d30" distance of L13 A5.centre
  measures "d31" distance of L15 A5.centre
  measures "d32" distance of L14 A5.centre
  measures "d33" diameter of A6
  measures "d34" diameter of A7
  measures "d35" distance of L23 A7.centre
  measures "d36" distance of L22 A7.centre
  measures "d37" distance of L20 A7.centre
  measures "d38" distance of L21 A7.centre
  measures "d39" distance of L17 A6.centre
  measures "d40" distance of L19 A6.centre
  measures "d41" distance of L18 A6.centre
  measures "d42" distance of L16 A6.centre
extrude "Extrude5" add sketch "Sketch5" against normal blind 6 contours L0 L3 A3 L16 L17 L18 L19 | A3 L18 L19 | L0 A0 L1 L12 L13 L14 L15 | A0 L12 L13 | L2 A2 L3 L20 L21 L22 L23 | A2 L22 L23 | L1 A1 L2 L8 L9 L10 L11 | A1 L8 L9 | A4 | A5 | A6 | A7
extrude "Extrude6" cut sketch "Sketch5" against normal blind 1.5 contours A4 | A5 | A6 | A7
fillet "Fillet3" radius 8 4 edges at (164, -3, 147) (164, -3, 47) (64, -3, 47) (64, -3, 147)
sketch "Sketch6" plane through (0, -25, 0) normal (0, 1, 0) x (-1, 0, 0)
  arc A0 (-52, 27) -> (-44, 35) centre (-52, 35) ccw
  line L0 (-44, 35) -> (-44, 159)
  arc A1 (-44, 159) -> (-52, 167) centre (-52, 159) ccw
  line L1 (-52, 167) -> (-176, 167)
  arc A2 (-176, 167) -> (-184, 159) centre (-176, 159) ccw
  line L2 (-184, 159) -> (-184, 35)
  arc A3 (-184, 35) -> (-176, 27) centre (-176, 35) ccw
  line L3 (-176, 27) -> (-52, 27)
  line L4 (-93, 128.5) -> (-60, 128.5)
  line L5 (-60, 128.5) -> (-60, 65.5)
  line L6 (-60, 65.5) -> (-93, 65.5)
  line L7 (-93, 65.5) -> (-93, 128.5)
  dimension "d51" = 63
  dimension "d54" = 33
  dimension "d88" = 16
  dimension "d92" = 38.5
  constraint horizontal L4
  constraint vertical L5
  constraint horizontal L6
  constraint vertical L7
  measures "d51" distance of L4.end L5.end
  measures "d54" distance of L4.start L4.end
  measures "d88" distance of L0 L5
  measures "d92" distance of L1 L4
extrude "Extrude7" cut sketch "Sketch6" against normal blind 4 contours L4 L5 L6 L7
sketch "Sketch7" plane through (0, -25, 0) normal (0, 1, 0) x (-1, 0, 0)
  line L0 (-60, 128.5) -> (-60, 65.5)
  line L1 (-60, 65.5) -> (-93, 65.5)
  line L2 (-93, 65.5) -> (-93, 128.5)
  line L3 (-93, 128.5) -> (-60, 128.5)
  arc A0 (-52, 27) -> (-44, 35) centre (-52, 35) ccw
  line L4 (-44, 35) -> (-44, 159)
  arc A1 (-44, 159) -> (-52, 167) centre (-52, 159) ccw
  line L5 (-52, 167) -> (-176, 167)
  arc A2 (-176, 167) -> (-184, 159) centre (-176, 159) ccw
  line L6 (-184, 159) -> (-184, 35)
  arc A3 (-184, 35) -> (-176, 27) centre (-176, 35) ccw
  line L7 (-176, 27) -> (-52, 27)
  line L8 (-96, 130.6162) -> (-99, 130.6162)
  line L9 (-99, 130.6162) -> (-99, 62.5)
  line L10 (-99, 62.5) -> (-96, 62.5)
  line L11 (-96, 62.5) -> (-96, 130.6162)
  line L12 (-96, 62.5) -> (-54, 62.5)
  line L13 (-54, 62.5) -> (-54, 65.5)
  line L14 (-54, 65.5) -> (-96, 65.5)
  line L15 (-96, 65.5) -> (-96, 62.5)
  line L16 (-54, 65.5) -> (-57, 65.5)
  line L17 (-57, 65.5) -> (-57, 130.6162)
  line L18 (-57, 130.6162) -> (-54, 130.6162)
  line L19 (-54, 130.6162) -> (-54, 65.5)
  dimension "d55" = 3
  dimension "d56" = 3
  dimension "d57" = 3
  dimension "d58" = 3
  dimension "d59" = 3
  constraint horizontal L8
  constraint vertical L9
  constraint horizontal L10
  constraint vertical L11
  constraint horizontal L12
  constraint vertical L13
  constraint horizontal L14
  constraint vertical L15
  constraint horizontal L16
  constraint vertical L17
  constraint horizontal L18
  constraint vertical L19
  constraint collinear L1 L14
  measures "d55" distance of L2 L11
  measures "d56" distance of L0 L17
  measures "d57" distance of L8.start L8.end
  measures "d58" distance of L17.end L18.end
  measures "d59" distance of L12.end L13.end
extrude "Extrude8" add sketch "Sketch7" along normal blind 4 contours L1 L11 L12 L13 L14 L15 L16 | L14 L16 L17 L18 L19 | L8 L9 L10 L11 L15
sketch "Sketch8" plane through (0, -25, 0) normal (0, 1, 0) x (-1, 0, 0)
  line L0 (-96, 65.5) -> (-93, 65.5)
  line L1 (-93, 65.5) -> (-93, 128.5)
  line L2 (-93, 128.5) -> (-60, 128.5)
  line L3 (-60, 128.5) -> (-60, 65.5)
  line L4 (-60, 65.5) -> (-57, 65.5)
  line L5 (-57, 65.5) -> (-57, 130.6162)
  line L6 (-57, 130.6162) -> (-54, 130.6162)
  line L7 (-54, 130.6162) -> (-54, 62.5)
  line L8 (-54, 62.5) -> (-99, 62.5)
  line L9 (-99, 62.5) -> (-99, 130.6162)
  line L10 (-99, 130.6162) -> (-96, 130.6162)
  line L11 (-96, 130.6162) -> (-96, 65.5)
  arc A0 (-52, 27) -> (-44, 35) centre (-52, 35) ccw
  line L12 (-44, 35) -> (-44, 159)
  arc A1 (-44, 159) -> (-52, 167) centre (-52, 159) ccw
  line L13 (-52, 167) -> (-176, 167)
  arc A2 (-176, 167) -> (-184, 159) centre (-176, 159) ccw
  line L14 (-184, 159) -> (-184, 35)
  arc A3 (-184, 35) -> (-176, 27) centre (-176, 35) ccw
  line L15 (-176, 27) -> (-52, 27)
  line L16 (-174, 142) -> (-144, 142)
  line L17 (-144, 142) -> (-144, 89)
  line L18 (-144, 89) -> (-174, 89)
  line L19 (-174, 89) -> (-174, 142)
  line L20 (-109, 142) -> (-139, 142)
  line L21 (-139, 142) -> (-139, 89)
  line L22 (-139, 89) -> (-109, 89)
  line L23 (-109, 89) -> (-109, 142)
  line L24 (-171.5, 84) -> (-111.5, 84)
  line L25 (-111.5, 84) -> (-111.5, 52)
  line L26 (-111.5, 52) -> (-171.5, 52)
  line L27 (-171.5, 52) -> (-171.5, 84)
  dimension "d60" = 30
  dimension "d61" = 53
  dimension "d64" = 30
  dimension "d65" = 53
  dimension "d66" = 60
  dimension "d67" = 32
  dimension "d86" = 5
  dimension "d87" = 25
  dimension "d89" = 10
  dimension "d90" = 5
  dimension "d91" = 2.5
  constraint horizontal L16
  constraint vertical L17
  constraint horizontal L18
  constraint vertical L19
  constraint horizontal L20
  constraint vertical L21
  constraint horizontal L22
  constraint vertical L23
  constraint horizontal L24
  constraint vertical L25
  constraint horizontal L26
  constraint vertical L27
  constraint collinear L16 L20
  measures "d60" distance of L16.start L16.end
  measures "d61" distance of L16.end L17.end
  measures "d64" distance of L20.start L20.end
  measures "d65" distance of L20.start L22.end
  measures "d66" distance of L24.start L24.end
  measures "d67" distance of L24.start L26.end
  measures "d86" distance of L22 L24
  measures "d87" distance of L13 L16
  measures "d89" distance of L9 L23
  measures "d90" distance of L17 L21
  measures "d91" distance of L19 L27
extrude "Extrude9" add sketch "Sketch8" along normal blind 2 contours L16 L17 L18 L19 | L20 L21 L22 L23 | L24 L25 L26 L27